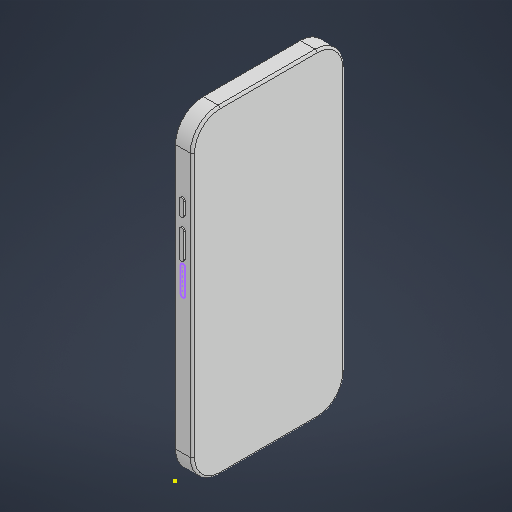
# Autodesk Inventor part: Peça1
Saved by Autodesk Inventor 2027.1 (Build 311270010, 270A)
## iProperties
Created: 2026-09-24
Part Number: Peça1
Material: Genérico
Document SubType Name: Modeling
Designer: labsfiap
Density: 1 g/cm^3
Appearance: Padrão
Author: labsfiap
Autodesk Inventor part; units mm, degrees
ref_plane "YZ Plane" through (0, 0, 0) normal (1, 0, 0) x (0, 1, 0)
ref_plane "XZ Plane" through (0, 0, 0) normal (0, 1, 0) x (-1, 0, 0)
ref_plane "XY Plane" through (0, 0, 0) normal (0, 0, 1) x (1, 0, 0)
sketch "Esboço1" plane through (0, 0, 0) normal (1, 0, 0) x (0, 1, 0)
  line L0 (0, 0) -> (149.6, 0)
  line L1 (149.6, 0) -> (149.6, -71.5)
  line L2 (149.6, -71.5) -> (0, -71.5)
  line L3 (0, -71.5) -> (0, 0)
  dimension "d0" = 149.6
  dimension "d1" = 71.5
  constraints: 8 end point, 3 perpendicular, 1 horizontal
  measures "d0" distance of L0.start L0.end
  measures "d1" distance of L0.end L1.end
extrude "Extrusão1" add sketch "Esboço1" along normal blind 7.95
fillet "Arredondamento1" radius 13 4 edges at (3.975, 149.6, -71.5) (3.975, 149.6, 0) (3.975, 0, 0) (3.975, 0, -71.5)
fillet "Arredondamento2" radius 1 8 edges at (7.95, 0, -35.75) (7.95, 3.8076, -67.6924) (7.95, 74.8, -71.5) (7.95, 145.7924, -67.6924) (7.95, 149.6, -35.75) (7.95, 145.7924, -3.8076) (7.95, 74.8, 0) (7.95, 3.8076, -3.8076)
sketch "Esboço2" plane through (0, 0, -58.5) normal (0, -1, 0) x (1, 0, 0)
  line L0 (6.95, 0) -> (0, 0) projected
  line L1 (0, 45.5) -> (6.95, 45.5) projected
  line L2 (3.475, 18.65) -> (4.775, 18.65)
  line L3 (4.775, 18.65) -> (2.175, 18.65)
  line L4 (2.175, 18.65) -> (2.175, 26.85)
  line L5 (2.175, 26.85) -> (4.775, 26.85)
  line L6 (4.775, 26.85) -> (4.775, 18.65)
  point P0 (0, 58.5)
  constraints: 10 end point, 3 perpendicular, 1 horizontal, 1 point on line
extrude "Extrusão2" cut sketch "Esboço2" against normal blind 6.2
fillet "Arredondamento3" radius 1.3 4 edges at (4.775, 3.1, -39.85) (2.175, 3.1, -39.85) (4.775, 3.1, -31.65) (2.175, 3.1, -31.65)
sketch "Esboço3" plane through (0, 6.2, -58.5) normal (0, -1, 0) x (1, 0, 0)
  arc A0 (4.775, 25.55) -> (2.175, 25.55) centre (3.475, 25.55) ccw projected
  arc A1 (2.175, 19.95) -> (4.775, 19.95) centre (3.475, 19.95) ccw projected
  line L0 (3.475, 25.55) -> (3.475, 19.95) construction
  line L1 (3.125, 25.55) -> (3.125, 19.95)
  line L2 (3.825, 19.95) -> (3.825, 25.55)
  arc A2 (3.825, 25.55) -> (3.125, 25.55) centre (3.475, 25.55) ccw
  arc A3 (3.125, 19.95) -> (3.825, 19.95) centre (3.475, 19.95) ccw
  point P0 (0, 58.5)
  point P1 (3.475, 22.75)
  constraints: 8 end point, 4 point on circle, 4 tangent, 2 centre point, 1 midpoint, 1 parallel
extrude "Extrusão3" add sketch "Esboço3" along normal blind 5.5
sketch "Esboço4" plane through (0, 0, 0) normal (-1, 0, 0) x (0, 0, 1)
  line L0 (-58.5, 149.6) -> (-13, 149.6) projected
  arc A0 (-58.5, 148.6) -> (-70.5, 136.6) centre (-58.5, 136.6) ccw projected
  line L1 (-66.5, 131.06) -> (-66.5, 110.31)
  line L2 (-45, 110.31) -> (-45, 131.06)
  arc A1 (-45, 131.06) -> (-66.5, 131.06) centre (-55.75, 131.06) ccw
  arc A2 (-66.5, 110.31) -> (-45, 110.31) centre (-55.75, 110.31) ccw
  circle A3 centre (-55.75, 131.06) radius 8.4
  circle A4 centre (-55.75, 131.06) radius 7.6
  circle A5 centre (-55.75, 131.06) radius 5.75
  circle A6 centre (-55.75, 110.31) radius 8.4
  circle A7 centre (-55.75, 110.31) radius 7.6
  circle A8 centre (-55.75, 110.31) radius 5.75
  point P0 (0, 0)
  constraints: 8 centre point, 6 coincident, 4 end point, 4 point on circle, 4 tangent, 1 parallel
extrude "Extrusão4" add sketch "Esboço4" along normal blind 2.2 contours A1 L2 A2 L1
sketch "Esboço5" plane through (0, 0, 0) normal (-1, 0, 0) x (0, 0, 1)
  circle A0 centre (-55.75, 131.06) radius 8.4 projected
  circle A1 centre (-55.75, 131.06) radius 7.6
  circle A2 centre (-55.75, 131.06) radius 5.75
  circle A3 centre (-55.75, 131.06) radius 8.4
  point P0 (0, 0)
  constraints: 3 centre point, 3 coincident, 1 concentric
extrude "Extrusão5" add sketch "Esboço5" along normal blind 3.3 contours A0
sketch "Esboço6" plane through (0, 131.06, -55.75) normal (-1, 0, 0) x (0, 0, 1)
  circle A0 centre (0, -20.75) radius 8.4 projected
  circle A1 centre (0, -20.75) radius 8.4
  circle A2 centre (0, -20.75) radius 7.6
  point P0 (55.75, -131.06)
  constraints: 2 centre point, 2 coincident
extrude "Extrusão6" add sketch "Esboço6" along normal blind 3.3
sketch "Esboço7" plane through (0, 131.06, -55.75) normal (-1, 0, 0) x (0, 0, 1)
  circle A0 centre (0, 0) radius 7.6
  circle A1 centre (0, -20.75) radius 7.6 projected
  circle A2 centre (0, -20.75) radius 7.6
  point P0 (55.75, -131.06)
  dimension "d38" = 15.2
  dimension "d40" = 15.2
  constraints: 2 centre point, 1 coincident
  measures "d38" diameter of A0
  measures "d40" diameter of A2
extrude "Extrusão7" add sketch "Esboço7" along normal blind 3.1
sketch "Esboço8" plane through (0, 0, 0) normal (-1, 0, 0) x (0, 0, 1)
  line L0 (-45, 110.31) -> (-45, 131.06) projected
  circle A0 centre (-35.7, 120.685) radius 2.5
  circle A1 centre (-35.7, 120.685) radius 2.3
  point P0 (0, 0)
  dimension "d45" = 4.6
  constraints: 2 centre point, 1 coincident
  measures "d45" diameter of A1
extrude "Extrusão8" add sketch "Esboço8" along normal blind 0.2 contours A0 | A1
sketch "Esboço9" plane through (0, 13, 0) normal (0, 0, 1) x (1, 0, 0)
  line L0 (0, 136.6) -> (6.95, 136.6) projected
  line L1 (2.375, 103) -> (2.375, 97.2)
  line L2 (4.575, 97.2) -> (4.575, 103)
  arc A0 (4.575, 103) -> (2.375, 103) centre (3.475, 103) ccw
  arc A1 (2.375, 97.2) -> (4.575, 97.2) centre (3.475, 97.2) ccw
  line L3 (3.475, 79.35) -> (3.475, 90.85) construction
  line L4 (4.575, 79.35) -> (4.575, 90.85)
  line L5 (2.375, 90.85) -> (2.375, 79.35)
  arc A2 (2.375, 79.35) -> (4.575, 79.35) centre (3.475, 79.35) ccw
  arc A3 (4.575, 90.85) -> (2.375, 90.85) centre (3.475, 90.85) ccw
  point P0 (0, -13)
  constraints: 12 end point, 8 point on circle, 8 tangent, 4 centre point, 2 parallel
sketch "Esboço10" plane through (0, 13, 0) normal (0, 0, 1) x (1, 0, 0)
  line L0 (3.4735, 64.3614) -> (3.4735, 75.8614) construction
  line L1 (4.5735, 64.3614) -> (4.5735, 75.8614)
  line L2 (2.3735, 75.8614) -> (2.3735, 64.3614)
  arc A0 (2.3735, 64.3614) -> (4.5735, 64.3614) centre (3.4735, 64.3614) ccw
  arc A1 (4.5735, 75.8614) -> (2.3735, 75.8614) centre (3.4735, 75.8614) ccw
  point P0 (0, -13)
  constraints: 8 end point, 4 point on circle, 4 tangent, 2 centre point, 1 parallel
extrude "Extrusão9" add sketch "Esboço9" along normal blind 0.6
